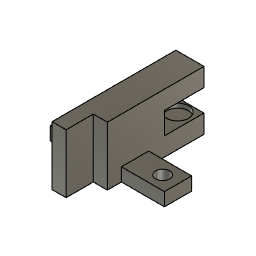
light_gate v4 (Autodesk Fusion 360 design; units mm, degrees)
Autodesk Fusion 360 part; units mm, degrees
note: some values were not read from the file. Set by a fixed rule: which sketch regions a step uses.
sketch "Sketch1" plane through (0, 0, 0) normal (0, 0, 1) x (1, 0, 0)
  line L0 (0, 0) -> (26, 0)
  line L1 (26, 0) -> (26, 6.2)
  line L2 (26, 6.2) -> (0, 6.2)
  line L3 (0, 6.2) -> (0, 0)
  dimension "d1" = 26
  dimension "d2" = 6.2
  constraint horizontal L0
  constraint vertical L1
  constraint horizontal L2
  constraint vertical L3
  constraint coincident L0.start L3.end
  measures "d1" distance of L0.start L0.end
  measures "d2" distance of L0.start L2.end
extrude "Extrude1" add sketch "Sketch1" along normal blind 3
sketch "Sketch2" plane through (0, 0, 0) normal (0, 0, 1) x (1, 0, 0)
  line L0 (0, 0) -> (13, 0)
  line L1 (13, 0) -> (13, -3.2)
  line L2 (13, -3.2) -> (9.8, -3.2)
  line L3 (9.8, -3.2) -> (9.8, 0)
  line L4 (9.8, 0) -> (13, 0)
  line L5 (13, 0) -> (13, -3.2)
  line L6 (13, -3.2) -> (16.2, -3.2)
  line L7 (16.2, -3.2) -> (16.2, 0)
  line L8 (16.2, 0) -> (13, 0)
  line L9 (13, 0) -> (13, -3.2)
  line L10 (9.8, -3.2) -> (16.2, -3.2)
  line L11 (16.2, -3.2) -> (16.2, 18.8)
  line L12 (16.2, 18.8) -> (9.8, 18.8)
  line L13 (9.8, 18.8) -> (9.8, -3.2)
  dimension "d5" = 13
  dimension "d6" = 3.2
  dimension "d7" = 3.2
  dimension "d8" = 3.2
  dimension "d9" = 6.4
  dimension "d10" = 22
  constraint coincident L0.start origin
  constraint horizontal L0
  constraint perpendicular L0 L1
  constraint horizontal L2
  constraint vertical L3
  constraint horizontal L4
  constraint vertical L5
  constraint coincident L0 L3.end
  constraint horizontal L6
  constraint vertical L7
  constraint horizontal L8
  constraint vertical L9
  constraint horizontal L10
  constraint vertical L11
  constraint horizontal L12
  constraint vertical L13
  measures "d5" distance of L0.start L0.end
  measures "d6" distance of L0.end L1.end
  measures "d7" distance of L1.end L2.end
  measures "d8" distance of L1.end L6.end
  measures "d9" distance of L2.end L6.end
  measures "d10" distance of L2.end L12.end
extrude "Extrude2" add sketch "Sketch2" along normal blind 13.4
sketch "Sketch3" plane through (0, -3.2, 0) normal (0, -1, 0) x (1, 0, 0)
  line L0 (9.8, 0) -> (16.2, 0)
  line L1 (16.2, 0) -> (16.2, 13.4)
  line L2 (16.2, 13.4) -> (9.8, 13.4)
  line L3 (9.8, 13.4) -> (9.8, 0)
  line L4 (9.8, 13.4) -> (13, 13.4)
  line L5 (13, 13.4) -> (13, 0)
  line L6 (13, 0) -> (9.8, 0)
  line L7 (9.8, 0) -> (9.8, 13.4)
  constraint horizontal L4
  constraint vertical L5
  constraint horizontal L6
  constraint vertical L7
  constraint midpoint L0 L5.end
  constraint coincident L2.end L3.start
extrude "Extrude3" add sketch "Sketch3" along normal blind 6.2 contours L0 L2 L3 L4 L5 L6 L7
sketch "Sketch4" plane through (0, 0, 3) normal (0, 0, 1) x (-1, 0, 0)
  line L0 (-9.8, 0) -> (-9.8, -6.2)
  line L1 (-9.8, -6.2) -> (0, -6.2)
  line L2 (0, -6.2) -> (0, 0)
  line L3 (0, 0) -> (-9.8, 0)
  line L4 (-13, 3) -> (-13, -19)
  line L5 (-13, -19) -> (-13, 3)
  line L6 (0, -3.1) -> (-26, -3.1)
  line L7 (-13, -3.1) -> (-3.5, -3.1)
  line L8 (-13, -3.1) -> (-22.5, -3.1)
  circle A0 centre (-3.5, -3.1) radius 1.6
  circle A1 centre (-22.5, -3.1) radius 1.6
  dimension "d15" = 9.5
  dimension "d16" = 9.5
  dimension "d17" = 3.2
  dimension "d18" = 3.2
  constraint perpendicular L1 L4
  constraint midpoint L2 L6.start
  constraint perpendicular L2 L6
  constraint midpoint L6 L7.start
  constraint perpendicular L5 L7
  constraint perpendicular L5 L8
  constraint coincident L7.end A0.centre
  constraint coincident L8.end A1.centre
  measures "d15" distance of L7.start L7.end
  measures "d16" distance of L7.start L8.end
  measures "d17" diameter of A0
  measures "d18" diameter of A1
extrude "Extrude4" cut sketch "Sketch4" against normal blind 17 contours L6 L7 A0 | L6 L7 A0 | L6 L8 A1 | L6 L8 A1
sketch "Sketch5" plane through (9.8, 0, 0) normal (-1, 0, 0) x (0, -1, 0)
  line L0 (-6.2, 0) -> (-6.2, 3)
  line L1 (-6.2, 3) -> (0, 3)
  line L2 (0, 3) -> (0, 0)
  line L3 (0, 0) -> (9.4, 0)
  line L4 (9.4, 0) -> (9.4, 13.4)
  line L5 (9.4, 13.4) -> (-18.8, 13.4)
  line L6 (-18.8, 13.4) -> (-18.8, 0)
  line L7 (-18.8, 0) -> (-6.2, 0)
  line L8 (-18.8, 6.7) -> (-9.8, 6.7)
  line L9 (-9.8, 6.7) -> (-9.8, 9.2)
  line L10 (-9.8, 9.2) -> (-18.8, 9.2)
  line L11 (-18.8, 9.2) -> (-18.8, 6.7)
  line L12 (-18.8, 6.7) -> (-9.8, 6.7)
  line L13 (-9.8, 6.7) -> (-9.8, 4.2)
  line L14 (-9.8, 4.2) -> (-18.8, 4.2)
  line L15 (-18.8, 4.2) -> (-18.8, 6.7)
  dimension "d21" = 9
  dimension "d22" = 2.5
  dimension "d23" = 2.5
  constraint horizontal L8
  constraint vertical L9
  constraint horizontal L10
  constraint vertical L11
  constraint midpoint L6 L8.start
  constraint horizontal L12
  constraint vertical L13
  constraint horizontal L14
  constraint vertical L15
  measures "d21" distance of L8.start L8.end
  measures "d22" distance of L8.start L10.end
  measures "d23" distance of L8.start L14.end
extrude "Extrude5" cut sketch "Sketch5" against normal blind 17 contours L6 L8 L12 L13 L14 L15 | L6 L8 L9 L10 L11 L12
sketch "Sketch6" plane through (0, 0, 4.2) normal (0, 0, 1) x (-1, 0, 0)
  line L0 (-16.2, -9.8) -> (-16.2, -18.8)
  line L1 (-16.2, -18.8) -> (-9.8, -18.8)
  line L2 (-9.8, -18.8) -> (-9.8, -9.8)
  line L3 (-9.8, -9.8) -> (-16.2, -9.8)
  line L4 (-13, -3) -> (-13, -16)
  circle A0 centre (-13, -16) radius 2.5
  dimension "d26" = 13
  dimension "d27" = 5
  constraint perpendicular L3 L4
  constraint coincident L4.end A0.centre
  measures "d26" distance of L4.start L4.end
  measures "d27" diameter of A0
extrude "Extrude6" cut sketch "Sketch6" against normal blind 1 contours A0
